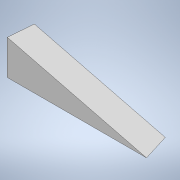
# Autodesk Inventor part: Domino ramp
Saved by Autodesk Inventor 2021 (Build 250183000, 183)
## iProperties
Created: 2021-02-17
Part Number: Domino ramp
Material: Generic
Document SubType Name: Modeling
Designer: david
Density: 1 g/cm^3
Appearance: Default
Author: david
Autodesk Inventor part; units mm, degrees
ref_plane "YZ Plane" through (0, 0, 0) normal (1, 0, 0) x (0, 1, 0)
ref_plane "XZ Plane" through (0, 0, 0) normal (0, 1, 0) x (-1, 0, 0)
ref_plane "XY Plane" through (0, 0, 0) normal (0, 0, 1) x (1, 0, 0)
sketch "Sketch1" plane through (0, 0, 0) normal (0, 0, 1) x (1, 0, 0)
  line L0 (21.7714, 74.3857) -> (21.7714, 10.8857)
  line L1 (21.7714, 10.8857) -> (275.7714, 10.8857)
  line L2 (275.7714, 10.8857) -> (21.7714, 74.3857)
  point P0 (0, 0)
  dimension "d0" = 63.5
  dimension "d1" = 254
  constraints: 6 end point, 1 vertical
  measures "d0" distance of L0.start L0.end
  measures "d1" distance of L0.end L1.end
extrude "Extrusion1" add sketch "Sketch1" along normal blind 50.8 draft 2
body "Solid1"
